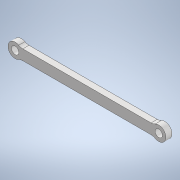
# Autodesk Inventor part: ff2
Saved by Autodesk Inventor 2020 (Build 240168000, 168)
## iProperties
Created: 2020-11-09
Part Number: ff2
Material: Generic
Document SubType Name: Modeling
Designer: alnwlsn
Density: 1 g/cm^3
Appearance: Default
Author: alnwlsn
Autodesk Inventor part; units mm, degrees
ref_plane "YZ Plane" through (0, 0, 0) normal (1, 0, 0) x (0, 1, 0)
ref_plane "XZ Plane" through (0, 0, 0) normal (0, 1, 0) x (-1, 0, 0)
ref_plane "XY Plane" through (0, 0, 0) normal (0, 0, 1) x (1, 0, 0)
sketch "Sketch1" plane through (0, 0, 0) normal (0, 0, 1) x (1, 0, 0)
  circle A0 centre (0, 0) radius 0.9
  circle A1 centre (0, 0) radius 1.75
  line L0 (0, 0) -> (32.6, 0) construction
  circle A2 centre (32.6, 0) radius 1.75
  circle A3 centre (32.6, 0) radius 0.9
  line L1 (0.9, 1.25) -> (31.7, 1.25)
  line L2 (31.7, 1.25) -> (31.7, -1.25)
  line L3 (31.7, -1.25) -> (0.9, -1.25)
  line L4 (0.9, -1.25) -> (0.9, 1.25)
  line L5 (0.9, 1.25) -> (31.7, -1.25) construction
  line L6 (31.7, 1.25) -> (0.9, -1.25) construction
  point P0 (16.3, 0)
  point P1 (1.2247, -1.25)
  point P2 (31.3753, -1.25)
  point P3 (31.3753, 1.25)
  point P4 (1.2247, 1.25)
  dimension "d0" = 1.8
  dimension "d1" = 3.5
  dimension "d8" = 2.5
  dimension "d9" = 32.6
  constraints: 14 end point, 4 centre point, 4 coincident, 3 midpoint, 2 equal radius, 2 horizontal, 2 parallel, 1 perpendicular, 1 tangent
  measures "d0" diameter of A0
  measures "d1" diameter of A1
  measures "d8" distance between parallel lines of L3 L1
  measures "d9" distance of point (0, 0) L0.end
extrude "Extrusion1" add sketch "Sketch1" along normal blind 1.5
fillet "Fillet2" radius 2 4 edges at (1.2247, 1.25, 0.75) (31.3753, 1.25, 0.75) (31.3753, -1.25, 0.75) (1.2247, -1.25, 0.75)
body "Solid1"
